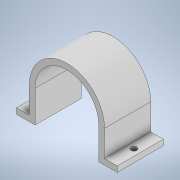
# Autodesk Inventor part: ShootingMech_MotorMount
Saved by Autodesk Inventor 2020 (Build 240168000, 168)
## iProperties
Created: 2022-01-28
Part Number: ShootingMech_MotorMount
Material: Generic
Document SubType Name: Modeling
Designer: danie
Density: 1 g/cm^3
Appearance: Default
Author: danie
Autodesk Inventor part; units mm, degrees
ref_plane "YZ Plane" through (0, 0, 0) normal (1, 0, 0) x (0, 1, 0)
ref_plane "XZ Plane" through (0, 0, 0) normal (0, 1, 0) x (-1, 0, 0)
ref_plane "XY Plane" through (0, 0, 0) normal (0, 0, 1) x (1, 0, 0)
sketch "Sketch1" plane through (0, 0, 0) normal (0, 0, 1) x (1, 0, 0)
  arc A0 (17.526, 0) -> (-17.526, 0) centre (0, 0) ccw
  arc A1 (20.701, 0) -> (-20.701, 0) centre (0, 0) ccw
  line L0 (17.526, 0) -> (20.701, 0)
  line L1 (20.701, 0) -> (20.701, -17.526)
  line L2 (20.701, -17.526) -> (17.526, -17.526)
  line L3 (17.526, -17.526) -> (17.526, 0)
  line L4 (-20.701, 0) -> (-17.526, 0)
  line L5 (-17.526, 0) -> (-17.526, -17.526)
  line L6 (-17.526, -17.526) -> (-20.701, -17.526)
  line L7 (-20.701, -17.526) -> (-20.701, 0)
  line L8 (-17.526, -17.526) -> (-27.686, -17.526)
  line L9 (-27.686, -17.526) -> (-27.686, -14.351)
  line L10 (-27.686, -14.351) -> (-17.526, -14.351)
  line L11 (-17.526, -14.351) -> (-17.526, -17.526)
  line L12 (17.526, -17.526) -> (27.686, -17.526)
  line L13 (27.686, -17.526) -> (27.686, -14.351)
  line L14 (27.686, -14.351) -> (17.526, -14.351)
  line L15 (17.526, -14.351) -> (17.526, -17.526)
  point P0 (-20.701, -14.351)
  point P1 (20.701, -14.351)
  dimension "d0" = 17.526
  dimension "d1" = 3.175
  dimension "d23" = 3.175
  dimension "d24" = 17.526
  dimension "d25" = 3.175
  dimension "d26" = 17.526
  dimension "d27" = 10.16
  dimension "d28" = 3.175
  dimension "d29" = 10.16
  dimension "d30" = 3.175
  constraints: 32 end point, 8 parallel, 4 horizontal, 4 perpendicular, 4 point on circle, 2 centre point, 1 coincident
  measures "d0" radius of A0
  measures "d1" radial gap between concentric circles of A0 A1
  measures "d23" distance of L1.end L2.end
  measures "d24" distance of L0.end L1.end
  measures "d25" distance of L5.end L6.end
  measures "d26" distance of L4.end L5.end
  measures "d27" distance of L9.end L10.end
  measures "d28" distance of L8.end L9.end
  measures "d29" distance of L14.end L13.end
  measures "d30" distance of L13.end L12.end
extrude "Extrusion1" add sketch "Sketch1" along normal blind 25.4
sketch "Sketch5" plane through (-27.686, -14.351, 0) normal (0, 1, 0) x (1, 0, 0)
  line L0 (6.985, 0) -> (0, 0) construction
  line L1 (6.985, -25.4) -> (0, -25.4) construction
  line L2 (0, 0) -> (6.985, -25.4) construction
  line L3 (0, 0) -> (0, -25.4) construction
  line L4 (6.985, 0) -> (0, -25.4) construction
  line L5 (45.212, -25.4) -> (55.372, -25.4) construction
  line L6 (48.387, 0) -> (55.372, -25.4) construction
  line L7 (45.212, 0) -> (55.372, 0) construction
  line L8 (55.372, 0) -> (48.387, -25.4) construction
  point P0 (27.686, 0)
  point P1 (3.4925, -12.7)
  constraints: 8 end point
sketch "Sketch6" plane through (20.701, -14.351, 0) normal (0, 1, 0) x (1, 0, 0)
  point P0 (-20.701, 0)
  point P1 (3.4926, -12.7006)
hole "Hole3" at (24.1936, -14.351, 12.7006) direction (0, -1, 0) diameter 3.175 end through all
hole "Hole4" at (-24.1935, -14.351, 12.7) direction (0, -1, 0) diameter 3.175 end through all
body "Solid1"
